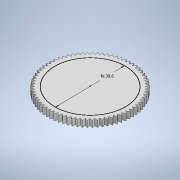
# Autodesk Inventor part: ChocolateCoin
Saved by Autodesk Inventor 2022.2 (Build 262287000, 287)
## iProperties
Created: 2022-07-18
Part Number: ChocolateCoin
Material: Generic
Document SubType Name: Modeling
Designer: ABL
Density: 1 g/cm^3
Appearance: Default
Author: ABL
Autodesk Inventor part; units mm, degrees
ref_plane "YZ Plane" through (0, 0, 0) normal (1, 0, 0) x (0, 1, 0)
ref_plane "XZ Plane" through (0, 0, 0) normal (0, 1, 0) x (-1, 0, 0)
ref_plane "XY Plane" through (0, 0, 0) normal (0, 0, 1) x (1, 0, 0)
sketch "Sketch1" plane through (0, 0, 0) normal (0, 1, 0) x (-1, 0, 0)
  circle A0 centre (0, 0) radius 22 construction
  line L0 (0, 0) -> (0, -22) construction
  line L1 (0, 0) -> (1.9174, -21.9163) construction
  line L2 (0, 0) -> (22, 0) construction
  line L3 (1.9174, -21.9163) -> (0, -22) construction
  line L4 (0, -22) -> (1.9174, -21.9163) construction
  line L5 (1.9174, -21.9163) -> (1.0312, -23.6187)
  line L6 (1.0312, -23.6187) -> (0, -22)
  line L7 (3.8203, -21.6658) -> (3.0858, -23.4389)
  line L8 (3.0858, -23.4389) -> (1.9174, -21.9163)
  line L9 (5.694, -21.2504) -> (5.1169, -23.0808)
  line L10 (5.1169, -23.0808) -> (3.8203, -21.6658)
  line L11 (7.5244, -20.6732) -> (7.109, -22.547)
  line L12 (7.109, -22.547) -> (5.694, -21.2504)
  line L13 (9.2976, -19.9388) -> (9.0471, -21.8416)
  line L14 (9.0471, -21.8416) -> (7.5244, -20.6732)
  line L15 (11, -19.0526) -> (10.9163, -20.97)
  line L16 (10.9163, -20.97) -> (9.2976, -19.9388)
  line L17 (12.6187, -18.0213) -> (12.7024, -19.9388)
  line L18 (12.7024, -19.9388) -> (11, -19.0526)
  line L19 (14.1413, -16.853) -> (14.3918, -18.7558)
  line L20 (14.3918, -18.7558) -> (12.6187, -18.0213)
  line L21 (15.5563, -15.5563) -> (15.9718, -17.4301)
  line L22 (15.9718, -17.4301) -> (14.1413, -16.853)
  line L23 (16.853, -14.1413) -> (17.4301, -15.9718)
  line L24 (17.4301, -15.9718) -> (15.5563, -15.5563)
  line L25 (18.0213, -12.6187) -> (18.7558, -14.3918)
  line L26 (18.7558, -14.3918) -> (16.853, -14.1413)
  line L27 (19.0526, -11) -> (19.9388, -12.7024)
  line L28 (19.9388, -12.7024) -> (18.0213, -12.6187)
  line L29 (19.9388, -9.2976) -> (20.97, -10.9163)
  line L30 (20.97, -10.9163) -> (19.0526, -11)
  line L31 (20.6732, -7.5244) -> (21.8416, -9.0471)
  line L32 (21.8416, -9.0471) -> (19.9388, -9.2976)
  line L33 (21.2504, -5.694) -> (22.547, -7.109)
  line L34 (22.547, -7.109) -> (20.6732, -7.5244)
  line L35 (21.6658, -3.8203) -> (23.0808, -5.1169)
  line L36 (23.0808, -5.1169) -> (21.2504, -5.694)
  line L37 (21.9163, -1.9174) -> (23.4389, -3.0858)
  line L38 (23.4389, -3.0858) -> (21.6658, -3.8203)
  line L39 (22, 0) -> (23.6187, -1.0312)
  line L40 (23.6187, -1.0312) -> (21.9163, -1.9174)
  line L41 (21.9163, 1.9174) -> (23.6187, 1.0312)
  line L42 (23.6187, 1.0312) -> (22, 0)
  line L43 (21.6658, 3.8203) -> (23.4389, 3.0858)
  line L44 (23.4389, 3.0858) -> (21.9163, 1.9174)
  line L45 (21.2504, 5.694) -> (23.0808, 5.1169)
  line L46 (23.0808, 5.1169) -> (21.6658, 3.8203)
  line L47 (20.6732, 7.5244) -> (22.547, 7.109)
  line L48 (22.547, 7.109) -> (21.2504, 5.694)
  line L49 (19.9388, 9.2976) -> (21.8416, 9.0471)
  line L50 (21.8416, 9.0471) -> (20.6732, 7.5244)
  line L51 (19.0526, 11) -> (20.97, 10.9163)
  line L52 (20.97, 10.9163) -> (19.9388, 9.2976)
  line L53 (18.0213, 12.6187) -> (19.9388, 12.7024)
  line L54 (19.9388, 12.7024) -> (19.0526, 11)
  line L55 (16.853, 14.1413) -> (18.7558, 14.3918)
  line L56 (18.7558, 14.3918) -> (18.0213, 12.6187)
  line L57 (15.5563, 15.5563) -> (17.4301, 15.9718)
  line L58 (17.4301, 15.9718) -> (16.853, 14.1413)
  line L59 (14.1413, 16.853) -> (15.9718, 17.4301)
  line L60 (15.9718, 17.4301) -> (15.5563, 15.5563)
  line L61 (12.6187, 18.0213) -> (14.3918, 18.7558)
  line L62 (14.3918, 18.7558) -> (14.1413, 16.853)
  line L63 (11, 19.0526) -> (12.7024, 19.9388)
  line L64 (12.7024, 19.9388) -> (12.6187, 18.0213)
  line L65 (9.2976, 19.9388) -> (10.9163, 20.97)
  line L66 (10.9163, 20.97) -> (11, 19.0526)
  line L67 (7.5244, 20.6732) -> (9.0471, 21.8416)
  line L68 (9.0471, 21.8416) -> (9.2976, 19.9388)
  line L69 (5.694, 21.2504) -> (7.109, 22.547)
  line L70 (7.109, 22.547) -> (7.5244, 20.6732)
  line L71 (3.8203, 21.6658) -> (5.1169, 23.0808)
  line L72 (5.1169, 23.0808) -> (5.694, 21.2504)
  line L73 (1.9174, 21.9163) -> (3.0858, 23.4389)
  line L74 (3.0858, 23.4389) -> (3.8203, 21.6658)
  line L75 (0, 22) -> (1.0312, 23.6187)
  line L76 (1.0312, 23.6187) -> (1.9174, 21.9163)
  line L77 (-1.9174, 21.9163) -> (-1.0312, 23.6187)
  line L78 (-1.0312, 23.6187) -> (0, 22)
  line L79 (-3.8203, 21.6658) -> (-3.0858, 23.4389)
  line L80 (-3.0858, 23.4389) -> (-1.9174, 21.9163)
  line L81 (-5.694, 21.2504) -> (-5.1169, 23.0808)
  line L82 (-5.1169, 23.0808) -> (-3.8203, 21.6658)
  line L83 (-7.5244, 20.6732) -> (-7.109, 22.547)
  line L84 (-7.109, 22.547) -> (-5.694, 21.2504)
  line L85 (-9.2976, 19.9388) -> (-9.0471, 21.8416)
  line L86 (-9.0471, 21.8416) -> (-7.5244, 20.6732)
  line L87 (-11, 19.0526) -> (-10.9163, 20.97)
  line L88 (-10.9163, 20.97) -> (-9.2976, 19.9388)
  line L89 (-12.6187, 18.0213) -> (-12.7024, 19.9388)
  line L90 (-12.7024, 19.9388) -> (-11, 19.0526)
  line L91 (-14.1413, 16.853) -> (-14.3918, 18.7558)
  line L92 (-14.3918, 18.7558) -> (-12.6187, 18.0213)
  line L93 (-15.5563, 15.5563) -> (-15.9718, 17.4301)
  line L94 (-15.9718, 17.4301) -> (-14.1413, 16.853)
  line L95 (-16.853, 14.1413) -> (-17.4301, 15.9718)
  line L96 (-17.4301, 15.9718) -> (-15.5563, 15.5563)
  line L97 (-18.0213, 12.6187) -> (-18.7558, 14.3918)
  line L98 (-18.7558, 14.3918) -> (-16.853, 14.1413)
  line L99 (-19.0526, 11) -> (-19.9388, 12.7024)
  line L100 (-19.9388, 12.7024) -> (-18.0213, 12.6187)
  line L101 (-19.9388, 9.2976) -> (-20.97, 10.9163)
  line L102 (-20.97, 10.9163) -> (-19.0526, 11)
  line L103 (-20.6732, 7.5244) -> (-21.8416, 9.0471)
  line L104 (-21.8416, 9.0471) -> (-19.9388, 9.2976)
  line L105 (-21.2504, 5.694) -> (-22.547, 7.109)
  line L106 (-22.547, 7.109) -> (-20.6732, 7.5244)
  line L107 (-21.6658, 3.8203) -> (-23.0808, 5.1169)
  line L108 (-23.0808, 5.1169) -> (-21.2504, 5.694)
  line L109 (-21.9163, 1.9174) -> (-23.4389, 3.0858)
  line L110 (-23.4389, 3.0858) -> (-21.6658, 3.8203)
  line L111 (-22, 0) -> (-23.6187, 1.0312)
  line L112 (-23.6187, 1.0312) -> (-21.9163, 1.9174)
  line L113 (-21.9163, -1.9174) -> (-23.6187, -1.0312)
  line L114 (-23.6187, -1.0312) -> (-22, 0)
  line L115 (-21.6658, -3.8203) -> (-23.4389, -3.0858)
  line L116 (-23.4389, -3.0858) -> (-21.9163, -1.9174)
  line L117 (-21.2504, -5.694) -> (-23.0808, -5.1169)
  line L118 (-23.0808, -5.1169) -> (-21.6658, -3.8203)
  line L119 (-20.6732, -7.5244) -> (-22.547, -7.109)
  line L120 (-22.547, -7.109) -> (-21.2504, -5.694)
  line L121 (-19.9388, -9.2976) -> (-21.8416, -9.0471)
  line L122 (-21.8416, -9.0471) -> (-20.6732, -7.5244)
  line L123 (-19.0526, -11) -> (-20.97, -10.9163)
  line L124 (-20.97, -10.9163) -> (-19.9388, -9.2976)
  line L125 (-18.0213, -12.6187) -> (-19.9388, -12.7024)
  line L126 (-19.9388, -12.7024) -> (-19.0526, -11)
  line L127 (-16.853, -14.1413) -> (-18.7558, -14.3918)
  line L128 (-18.7558, -14.3918) -> (-18.0213, -12.6187)
  line L129 (-15.5563, -15.5563) -> (-17.4301, -15.9718)
  line L130 (-17.4301, -15.9718) -> (-16.853, -14.1413)
  line L131 (-14.1413, -16.853) -> (-15.9718, -17.4301)
  line L132 (-15.9718, -17.4301) -> (-15.5563, -15.5563)
  line L133 (-12.6187, -18.0213) -> (-14.3918, -18.7558)
  line L134 (-14.3918, -18.7558) -> (-14.1413, -16.853)
  line L135 (-11, -19.0526) -> (-12.7024, -19.9388)
  line L136 (-12.7024, -19.9388) -> (-12.6187, -18.0213)
  line L137 (-9.2976, -19.9388) -> (-10.9163, -20.97)
  line L138 (-10.9163, -20.97) -> (-11, -19.0526)
  line L139 (-7.5244, -20.6732) -> (-9.0471, -21.8416)
  line L140 (-9.0471, -21.8416) -> (-9.2976, -19.9388)
  line L141 (-5.694, -21.2504) -> (-7.109, -22.547)
  line L142 (-7.109, -22.547) -> (-7.5244, -20.6732)
  line L143 (-3.8203, -21.6658) -> (-5.1169, -23.0808)
  line L144 (-5.1169, -23.0808) -> (-5.694, -21.2504)
  line L145 (-1.9174, -21.9163) -> (-3.0858, -23.4389)
  line L146 (-3.0858, -23.4389) -> (-3.8203, -21.6658)
  line L147 (0, -22) -> (-1.0312, -23.6187)
  line L148 (-1.0312, -23.6187) -> (-1.9174, -21.9163)
  point P0 (0.9829, -22.5117)
  dimension "d0" = 44
  dimension "d1" = 22
  dimension "d2" = 85
  dimension "d5" = 360
  constraints: 298 end point, 1 coincident, 1 equal length, 1 horizontal, 1 vertical, 1 vertical alignment, 370 other
  measures "d1" distance of L0.start L1.end
  measures "d2" angle of L1 L2
extrude "Extrusion1" add sketch "Sketch1" along normal blind 3.5
sketch "Sketch2" plane through (0, 3.5, 0) normal (0, 1, 0) x (1, 0, 0)
  circle A0 centre (0, 0) radius 19.8
  dimension "d9" = 39.6
  constraints: 1 centre point, 1 coincident
  measures "d9" diameter of A0
equation "\"d9\" = 0.9 * d0"
body "Solid1"
